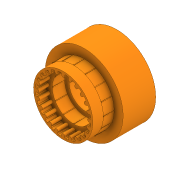
# Autodesk Inventor part: 4th Axis Barrel
Saved by Autodesk Inventor 2020 (Build 240168000, 168)
## iProperties
Created: 2021-06-26
Part Number: 4th Axis Barrel
Material: Generic
Document SubType Name: Modeling
Designer: Coy
Density: 1 g/cm^3
Appearance: Orange
Author: Coy
Autodesk Inventor part; units mm, degrees
ref_plane "YZ Plane" through (0, 0, 0) normal (1, 0, 0) x (0, 1, 0)
ref_plane "XZ Plane" through (0, 0, 0) normal (0, 1, 0) x (-1, 0, 0)
ref_plane "XY Plane" through (0, 0, 0) normal (0, 0, 1) x (1, 0, 0)
sketch "Sketch1" plane through (0, 0, 0) normal (0, 0, 1) x (1, 0, 0)
  circle A0 centre (0, 0) radius 11
  circle A1 centre (0, 0) radius 26
  dimension "d0" = 22
  dimension "d1" = 52
  constraints: 2 centre point, 2 coincident
  measures "d0" diameter of A0
  measures "d1" diameter of A1
extrude "Extrusion1" add sketch "Sketch1" against normal blind 21.75
sketch "Sketch2" plane through (0, 0, 0) normal (0, 0, 1) x (1, 0, 0)
  circle A0 centre (0, 0) radius 14
  circle A1 centre (0, 0) radius 20
  dimension "d4" = 28
  dimension "d5" = 40
  constraints: 2 centre point, 2 coincident
  measures "d4" diameter of A0
  measures "d5" diameter of A1
extrude "Extrusion2" add sketch "Sketch2" along normal blind 7
chamfer "Chamfer2" distance 7 angle 2 1 edges at (-20, 0, 7) measured on face at (-20, 0, 6.5)
sketch "Sketch4" plane through (0, 0, 7) normal (0, 0, 1) x (1, 0, 0)
  circle A0 centre (0, 0) radius 20 construction
  circle A1 centre (0, 0) radius 19.7556 projected
  arc A2 (0.2, 19.999) -> (-0.2, 19.999) centre (0, 20) ccw
  line L0 (-0.2, 19.999) -> (-0.1988, 19.7546)
  line L1 (0.2, 19.999) -> (0.1988, 19.7546)
  arc A3 (-7.4685, 18.5532) -> (-7.8381, 18.4001) centre (-7.6537, 18.4776) ccw
  line L2 (-7.8381, 18.4001) -> (-7.7434, 18.1748)
  line L3 (-7.4685, 18.5532) -> (-7.3761, 18.3269)
  arc A4 (-14, 14.2828) -> (-14.2828, 14) centre (-14.1421, 14.1421) ccw
  line L4 (-14.2828, 14) -> (-14.1091, 13.828)
  line L5 (-14, 14.2828) -> (-13.828, 14.1091)
  arc A5 (-18.4001, 7.8381) -> (-18.5532, 7.4685) centre (-18.4776, 7.6537) ccw
  line L6 (-18.5532, 7.4685) -> (-18.3269, 7.3761)
  line L7 (-18.4001, 7.8381) -> (-18.1748, 7.7434)
  arc A6 (-19.999, 0.2) -> (-19.999, -0.2) centre (-20, 0) ccw
  line L8 (-19.999, -0.2) -> (-19.7546, -0.1988)
  line L9 (-19.999, 0.2) -> (-19.7546, 0.1988)
  arc A7 (-18.5532, -7.4685) -> (-18.4001, -7.8381) centre (-18.4776, -7.6537) ccw
  line L10 (-18.4001, -7.8381) -> (-18.1748, -7.7434)
  line L11 (-18.5532, -7.4685) -> (-18.3269, -7.3761)
  arc A8 (-14.2828, -14) -> (-14, -14.2828) centre (-14.1421, -14.1421) ccw
  line L12 (-14, -14.2828) -> (-13.828, -14.1091)
  line L13 (-14.2828, -14) -> (-14.1091, -13.828)
  arc A9 (-7.8381, -18.4001) -> (-7.4685, -18.5532) centre (-7.6537, -18.4776) ccw
  line L14 (-7.4685, -18.5532) -> (-7.3761, -18.3269)
  line L15 (-7.8381, -18.4001) -> (-7.7434, -18.1748)
  arc A10 (-0.2, -19.999) -> (0.2, -19.999) centre (0, -20) ccw
  line L16 (0.2, -19.999) -> (0.1988, -19.7546)
  line L17 (-0.2, -19.999) -> (-0.1988, -19.7546)
  arc A11 (7.4685, -18.5532) -> (7.8381, -18.4001) centre (7.6537, -18.4776) ccw
  line L18 (7.8381, -18.4001) -> (7.7434, -18.1748)
  line L19 (7.4685, -18.5532) -> (7.3761, -18.3269)
  arc A12 (14, -14.2828) -> (14.2828, -14) centre (14.1421, -14.1421) ccw
  line L20 (14.2828, -14) -> (14.1091, -13.828)
  line L21 (14, -14.2828) -> (13.828, -14.1091)
  arc A13 (18.4001, -7.8381) -> (18.5532, -7.4685) centre (18.4776, -7.6537) ccw
  line L22 (18.5532, -7.4685) -> (18.3269, -7.3761)
  line L23 (18.4001, -7.8381) -> (18.1748, -7.7434)
  arc A14 (19.999, -0.2) -> (19.999, 0.2) centre (20, 0) ccw
  line L24 (19.999, 0.2) -> (19.7546, 0.1988)
  line L25 (19.999, -0.2) -> (19.7546, -0.1988)
  arc A15 (18.5532, 7.4685) -> (18.4001, 7.8381) centre (18.4776, 7.6537) ccw
  line L26 (18.4001, 7.8381) -> (18.1748, 7.7434)
  line L27 (18.5532, 7.4685) -> (18.3269, 7.3761)
  arc A16 (14.2828, 14) -> (14, 14.2828) centre (14.1421, 14.1421) ccw
  line L28 (14, 14.2828) -> (13.828, 14.1091)
  line L29 (14.2828, 14) -> (14.1091, 13.828)
  arc A17 (7.8381, 18.4001) -> (7.4685, 18.5532) centre (7.6537, 18.4776) ccw
  line L30 (7.4685, 18.5532) -> (7.3761, 18.3269)
  line L31 (7.8381, 18.4001) -> (7.7434, 18.1748)
  dimension "d25" = 0.4
  dimension "d28" = 360
  constraints: 64 end point, 35 point on circle, 16 centre point, 2 tangent, 132 other
  measures "d25" diameter of A2
extrude "Extrusion4" add sketch "Sketch4" against normal up to surface (7 mm away) contours A1 L24 A14 L25 | A1 L26 A15 L27 | L22 A13 L23 A1 | A1 L28 A16 L29 | L20 A12 L21 A1 | A1 L30 A17 L31 | L18 A11 L19 A1 | A1 L0 A2 L1 | L16 A10 L17 A1 | A1 L2 A3 L3 | L14 A9 L15 A1 | A1 L4 A4 L5 | L12 A8 L13 A1 | A1 L6 A5 L7 | L10 A7 L11 A1 | A1 L8 A6 L9
sketch "Sketch5" plane through (0, 0, 7) normal (0, 0, 1) x (1, 0, 0)
  arc A0 (7.3761, 18.3269) -> (0.1988, 19.7546) centre (0, 0) ccw projected
  arc A1 (-0.1988, 19.7546) -> (-7.3761, 18.3269) centre (0, 0) ccw projected
  circle A2 centre (0, 0) radius 19.7556
  line L0 (0, 0) -> (0, 34.6201) construction
  line L1 (1.1056, 17.9252) -> (1, 16.2136) construction
  line L2 (-1.1056, 17.9252) -> (-1, 16.2136) construction
  arc A3 (-1.0636, 17.2444) -> (1.0636, 17.2444) centre (0, 17.31) ccw
  line L3 (-1.0636, 17.2444) -> (-1.1056, 17.9252)
  line L4 (1.0636, 17.2444) -> (1.1056, 17.9252)
  arc A4 (1.6859, 18.423) -> (1.1056, 17.9252) centre (1.6374, 17.8924) ccw
  arc A5 (-1.1056, 17.9252) -> (-1.6859, 18.423) centre (-1.6374, 17.8924) ccw
  arc A6 (-5.7073, 17.0283) -> (-6.3967, 17.3589) centre (-6.2125, 16.859) ccw
  line L5 (-5.4905, 16.3816) -> (-5.7073, 17.0283)
  arc A7 (-5.4905, 16.3816) -> (-3.4359, 16.9321) centre (-4.4802, 16.7202) ccw
  line L6 (-3.4359, 16.9321) -> (-3.5715, 17.6006)
  arc A8 (-3.1398, 18.2316) -> (-3.5715, 17.6006) centre (-3.0493, 17.7065) ccw
  arc A9 (-9.9201, 14.9709) -> (-10.6715, 15.1119) centre (-10.3642, 14.6766) ccw
  line L7 (-9.5433, 14.4023) -> (-9.9201, 14.9709)
  arc A10 (-9.5433, 14.4023) -> (-7.7011, 15.4659) centre (-8.655, 14.9909) ccw
  line L8 (-7.7011, 15.4659) -> (-8.0052, 16.0765)
  arc A11 (-7.7515, 16.7978) -> (-8.0052, 16.0765) centre (-7.5282, 16.314) ccw
  arc A12 (-13.4568, 11.8933) -> (-14.2192, 11.8349) centre (-13.8096, 11.4941) ccw
  line L9 (-12.9457, 11.4416) -> (-13.4568, 11.8933)
  arc A13 (-12.9457, 11.4416) -> (-11.4416, 12.9457) centre (-12.24, 12.24) ccw
  line L10 (-11.4416, 12.9457) -> (-11.8933, 13.4568)
  arc A14 (-11.8349, 14.2192) -> (-11.8933, 13.4568) centre (-11.4941, 13.8096) ccw
  arc A15 (-16.0765, 8.0052) -> (-16.7978, 7.7515) centre (-16.314, 7.5282) ccw
  line L11 (-15.4659, 7.7011) -> (-16.0765, 8.0052)
  arc A16 (-15.4659, 7.7011) -> (-14.4023, 9.5433) centre (-14.9909, 8.655) ccw
  line L12 (-14.4023, 9.5433) -> (-14.9709, 9.9201)
  arc A17 (-15.1119, 10.6715) -> (-14.9709, 9.9201) centre (-14.6766, 10.3642) ccw
  arc A18 (-17.6006, 3.5715) -> (-18.2316, 3.1398) centre (-17.7065, 3.0493) ccw
  line L13 (-16.9321, 3.4359) -> (-17.6006, 3.5715)
  arc A19 (-16.9321, 3.4359) -> (-16.3816, 5.4905) centre (-16.7202, 4.4802) ccw
  line L14 (-16.3816, 5.4905) -> (-17.0283, 5.7073)
  arc A20 (-17.3589, 6.3967) -> (-17.0283, 5.7073) centre (-16.859, 6.2125) ccw
  arc A21 (-17.9252, -1.1056) -> (-18.423, -1.6859) centre (-17.8924, -1.6374) ccw
  line L15 (-17.2444, -1.0636) -> (-17.9252, -1.1056)
  arc A22 (-17.2444, -1.0636) -> (-17.2444, 1.0636) centre (-17.31, 0) ccw
  line L16 (-17.2444, 1.0636) -> (-17.9252, 1.1056)
  arc A23 (-18.423, 1.6859) -> (-17.9252, 1.1056) centre (-17.8924, 1.6374) ccw
  arc A24 (-17.0283, -5.7073) -> (-17.3589, -6.3967) centre (-16.859, -6.2125) ccw
  line L17 (-16.3816, -5.4905) -> (-17.0283, -5.7073)
  arc A25 (-16.3816, -5.4905) -> (-16.9321, -3.4359) centre (-16.7202, -4.4802) ccw
  line L18 (-16.9321, -3.4359) -> (-17.6006, -3.5715)
  arc A26 (-18.2316, -3.1398) -> (-17.6006, -3.5715) centre (-17.7065, -3.0493) ccw
  arc A27 (-14.9709, -9.9201) -> (-15.1119, -10.6715) centre (-14.6766, -10.3642) ccw
  line L19 (-14.4023, -9.5433) -> (-14.9709, -9.9201)
  arc A28 (-14.4023, -9.5433) -> (-15.4659, -7.7011) centre (-14.9909, -8.655) ccw
  line L20 (-15.4659, -7.7011) -> (-16.0765, -8.0052)
  arc A29 (-16.7978, -7.7515) -> (-16.0765, -8.0052) centre (-16.314, -7.5282) ccw
  arc A30 (-11.8933, -13.4568) -> (-11.8349, -14.2192) centre (-11.4941, -13.8096) ccw
  line L21 (-11.4416, -12.9457) -> (-11.8933, -13.4568)
  arc A31 (-11.4416, -12.9457) -> (-12.9457, -11.4416) centre (-12.24, -12.24) ccw
  line L22 (-12.9457, -11.4416) -> (-13.4568, -11.8933)
  arc A32 (-14.2192, -11.8349) -> (-13.4568, -11.8933) centre (-13.8096, -11.4941) ccw
  arc A33 (-8.0052, -16.0765) -> (-7.7515, -16.7978) centre (-7.5282, -16.314) ccw
  line L23 (-7.7011, -15.4659) -> (-8.0052, -16.0765)
  arc A34 (-7.7011, -15.4659) -> (-9.5433, -14.4023) centre (-8.655, -14.9909) ccw
  line L24 (-9.5433, -14.4023) -> (-9.9201, -14.9709)
  arc A35 (-10.6715, -15.1119) -> (-9.9201, -14.9709) centre (-10.3642, -14.6766) ccw
  arc A36 (-3.5715, -17.6006) -> (-3.1398, -18.2316) centre (-3.0493, -17.7065) ccw
  line L25 (-3.4359, -16.9321) -> (-3.5715, -17.6006)
  arc A37 (-3.4359, -16.9321) -> (-5.4905, -16.3816) centre (-4.4802, -16.7202) ccw
  line L26 (-5.4905, -16.3816) -> (-5.7073, -17.0283)
  arc A38 (-6.3967, -17.3589) -> (-5.7073, -17.0283) centre (-6.2125, -16.859) ccw
  arc A39 (1.1056, -17.9252) -> (1.6859, -18.423) centre (1.6374, -17.8924) ccw
  line L27 (1.0636, -17.2444) -> (1.1056, -17.9252)
  arc A40 (1.0636, -17.2444) -> (-1.0636, -17.2444) centre (0, -17.31) ccw
  line L28 (-1.0636, -17.2444) -> (-1.1056, -17.9252)
  arc A41 (-1.6859, -18.423) -> (-1.1056, -17.9252) centre (-1.6374, -17.8924) ccw
  arc A42 (5.7073, -17.0283) -> (6.3967, -17.3589) centre (6.2125, -16.859) ccw
  line L29 (5.4905, -16.3816) -> (5.7073, -17.0283)
  arc A43 (5.4905, -16.3816) -> (3.4359, -16.9321) centre (4.4802, -16.7202) ccw
  line L30 (3.4359, -16.9321) -> (3.5715, -17.6006)
  arc A44 (3.1398, -18.2316) -> (3.5715, -17.6006) centre (3.0493, -17.7065) ccw
  arc A45 (9.9201, -14.9709) -> (10.6715, -15.1119) centre (10.3642, -14.6766) ccw
  line L31 (9.5433, -14.4023) -> (9.9201, -14.9709)
  arc A46 (9.5433, -14.4023) -> (7.7011, -15.4659) centre (8.655, -14.9909) ccw
  line L32 (7.7011, -15.4659) -> (8.0052, -16.0765)
  arc A47 (7.7515, -16.7978) -> (8.0052, -16.0765) centre (7.5282, -16.314) ccw
  arc A48 (13.4568, -11.8933) -> (14.2192, -11.8349) centre (13.8096, -11.4941) ccw
  line L33 (12.9457, -11.4416) -> (13.4568, -11.8933)
  arc A49 (12.9457, -11.4416) -> (11.4416, -12.9457) centre (12.24, -12.24) ccw
  line L34 (11.4416, -12.9457) -> (11.8933, -13.4568)
  arc A50 (11.8349, -14.2192) -> (11.8933, -13.4568) centre (11.4941, -13.8096) ccw
  arc A51 (16.0765, -8.0052) -> (16.7978, -7.7515) centre (16.314, -7.5282) ccw
  line L35 (15.4659, -7.7011) -> (16.0765, -8.0052)
  arc A52 (15.4659, -7.7011) -> (14.4023, -9.5433) centre (14.9909, -8.655) ccw
  line L36 (14.4023, -9.5433) -> (14.9709, -9.9201)
  arc A53 (15.1119, -10.6715) -> (14.9709, -9.9201) centre (14.6766, -10.3642) ccw
  arc A54 (17.6006, -3.5715) -> (18.2316, -3.1398) centre (17.7065, -3.0493) ccw
  line L37 (16.9321, -3.4359) -> (17.6006, -3.5715)
  arc A55 (16.9321, -3.4359) -> (16.3816, -5.4905) centre (16.7202, -4.4802) ccw
  line L38 (16.3816, -5.4905) -> (17.0283, -5.7073)
  arc A56 (17.3589, -6.3967) -> (17.0283, -5.7073) centre (16.859, -6.2125) ccw
  arc A57 (17.9252, 1.1056) -> (18.423, 1.6859) centre (17.8924, 1.6374) ccw
  line L39 (17.2444, 1.0636) -> (17.9252, 1.1056)
  arc A58 (17.2444, 1.0636) -> (17.2444, -1.0636) centre (17.31, 0) ccw
  line L40 (17.2444, -1.0636) -> (17.9252, -1.1056)
  arc A59 (18.423, -1.6859) -> (17.9252, -1.1056) centre (17.8924, -1.6374) ccw
  arc A60 (17.0283, 5.7073) -> (17.3589, 6.3967) centre (16.859, 6.2125) ccw
  line L41 (16.3816, 5.4905) -> (17.0283, 5.7073)
  arc A61 (16.3816, 5.4905) -> (16.9321, 3.4359) centre (16.7202, 4.4802) ccw
  line L42 (16.9321, 3.4359) -> (17.6006, 3.5715)
  arc A62 (18.2316, 3.1398) -> (17.6006, 3.5715) centre (17.7065, 3.0493) ccw
  arc A63 (14.9709, 9.9201) -> (15.1119, 10.6715) centre (14.6766, 10.3642) ccw
  line L43 (14.4023, 9.5433) -> (14.9709, 9.9201)
  arc A64 (14.4023, 9.5433) -> (15.4659, 7.7011) centre (14.9909, 8.655) ccw
  line L44 (15.4659, 7.7011) -> (16.0765, 8.0052)
  arc A65 (16.7978, 7.7515) -> (16.0765, 8.0052) centre (16.314, 7.5282) ccw
  arc A66 (11.8933, 13.4568) -> (11.8349, 14.2192) centre (11.4941, 13.8096) ccw
  line L45 (11.4416, 12.9457) -> (11.8933, 13.4568)
  arc A67 (11.4416, 12.9457) -> (12.9457, 11.4416) centre (12.24, 12.24) ccw
  line L46 (12.9457, 11.4416) -> (13.4568, 11.8933)
  arc A68 (14.2192, 11.8349) -> (13.4568, 11.8933) centre (13.8096, 11.4941) ccw
  arc A69 (8.0052, 16.0765) -> (7.7515, 16.7978) centre (7.5282, 16.314) ccw
  line L47 (7.7011, 15.4659) -> (8.0052, 16.0765)
  arc A70 (7.7011, 15.4659) -> (9.5433, 14.4023) centre (8.655, 14.9909) ccw
  line L48 (9.5433, 14.4023) -> (9.9201, 14.9709)
  arc A71 (10.6715, 15.1119) -> (9.9201, 14.9709) centre (10.3642, 14.6766) ccw
  arc A72 (3.5715, 17.6006) -> (3.1398, 18.2316) centre (3.0493, 17.7065) ccw
  line L49 (3.4359, 16.9321) -> (3.5715, 17.6006)
  arc A73 (3.4359, 16.9321) -> (5.4905, 16.3816) centre (4.4802, 16.7202) ccw
  line L50 (5.4905, 16.3816) -> (5.7073, 17.0283)
  arc A74 (6.3967, 17.3589) -> (5.7073, 17.0283) centre (6.2125, 16.859) ccw
  arc A75 (-1.6859, 18.423) -> (-3.1398, 18.2316) centre (0, 0) ccw
  arc A76 (-6.3967, 17.3589) -> (-7.7515, 16.7978) centre (0, 0) ccw
  arc A77 (-10.6715, 15.1119) -> (-11.8349, 14.2192) centre (0, 0) ccw
  arc A78 (-14.2192, 11.8349) -> (-15.1119, 10.6715) centre (0, 0) ccw
  arc A79 (-16.7978, 7.7515) -> (-17.3589, 6.3967) centre (0, 0) ccw
  arc A80 (-18.2316, 3.1398) -> (-18.423, 1.6859) centre (0, 0) ccw
  arc A81 (-18.423, -1.6859) -> (-18.2316, -3.1398) centre (0, 0) ccw
  arc A82 (-17.3589, -6.3967) -> (-16.7978, -7.7515) centre (0, 0) ccw
  arc A83 (-15.1119, -10.6715) -> (-14.2192, -11.8349) centre (0, 0) ccw
  arc A84 (-11.8349, -14.2192) -> (-10.6715, -15.1119) centre (0, 0) ccw
  arc A85 (-7.7515, -16.7978) -> (-6.3967, -17.3589) centre (0, 0) ccw
  arc A86 (-3.1398, -18.2316) -> (-1.6859, -18.423) centre (0, 0) ccw
  arc A87 (1.6859, -18.423) -> (3.1398, -18.2316) centre (0, 0) ccw
  arc A88 (6.3967, -17.3589) -> (7.7515, -16.7978) centre (0, 0) ccw
  arc A89 (10.6715, -15.1119) -> (11.8349, -14.2192) centre (0, 0) ccw
  arc A90 (14.2192, -11.8349) -> (15.1119, -10.6715) centre (0, 0) ccw
  arc A91 (16.7978, -7.7515) -> (17.3589, -6.3967) centre (0, 0) ccw
  arc A92 (18.2316, -3.1398) -> (18.423, -1.6859) centre (0, 0) ccw
  arc A93 (18.423, 1.6859) -> (18.2316, 3.1398) centre (0, 0) ccw
  arc A94 (17.3589, 6.3967) -> (16.7978, 7.7515) centre (0, 0) ccw
  arc A95 (15.1119, 10.6715) -> (14.2192, 11.8349) centre (0, 0) ccw
  arc A96 (11.8349, 14.2192) -> (10.6715, 15.1119) centre (0, 0) ccw
  arc A97 (7.7515, 16.7978) -> (6.3967, 17.3589) centre (0, 0) ccw
  arc A98 (3.1398, 18.2316) -> (1.6859, 18.423) centre (0, 0) ccw
  circle A99 centre (0, 0) radius 16 construction
  point P0 (0.1988, 19.7546)
  point P1 (-7.3761, 18.3269)
  point P2 (7.3761, 18.3269)
  dimension "d33" = 1
  dimension "d38" = 1
  dimension "d40" = 1.0656
  dimension "d41" = 1.0656
  dimension "d42" = 1.0656
  dimension "d45" = 360
  dimension "d49" = 32
  constraints: 192 point on circle, 102 end point, 97 centre point, 4 coincident, 3 tangent, 2 line through centre, 2 point on line, 1 midpoint, 1 vertical, 340 other
  measures "d33" distance from line of L0 L2.end
  measures "d38" distance from line of L0 L1.end
  measures "d40" radius of A3
  measures "d41" diameter of A5
  measures "d42" diameter of A4
  measures "d49" diameter of A99
extrude "Extrusion5" add sketch "Sketch5" along normal blind 7
sketch "Sketch8" plane through (0, 0, 0) normal (0, 0, 1) x (1, 0, 0)
  circle A0 centre (0, 0) radius 14 projected
  circle A1 centre (0, 0) radius 11 projected
extrude "Extrusion7" cut sketch "Sketch8" against normal blind 1
chamfer "Chamfer4" distance 8 angle 2 1 edges at (-14, 0, 7) measured on face at (-14, 0, 6.5)
sketch "Sketch10" plane through (0, 0, 7) normal (0, 0, 1) x (1, 0, 0)
  circle A0 centre (0, 0) radius 14 construction
  circle A1 centre (0, 0) radius 14.2794 projected
  arc A2 (-0.2, 13.9986) -> (0.2, 13.9986) centre (0, 14) ccw
  line L0 (0.204, 14.2779) -> (0.2, 13.9971)
  line L1 (-0.204, 14.2779) -> (-0.2, 13.9971)
  line L2 (-7.3156, 12.263) -> (-7.1718, 12.0219)
  arc A3 (-7.1725, 12.0231) -> (-6.8261, 12.2231) centre (-7, 12.1244) ccw
  line L3 (-6.9623, 12.467) -> (-6.8254, 12.2219)
  line L4 (-12.467, 6.9623) -> (-12.2219, 6.8254)
  arc A4 (-12.2231, 6.8261) -> (-12.0231, 7.1725) centre (-12.1244, 7) ccw
  line L5 (-12.263, 7.3156) -> (-12.0219, 7.1718)
  line L6 (-14.2779, -0.204) -> (-13.9971, -0.2)
  arc A5 (-13.9986, -0.2) -> (-13.9986, 0.2) centre (-14, 0) ccw
  line L7 (-14.2779, 0.204) -> (-13.9971, 0.2)
  line L8 (-12.263, -7.3156) -> (-12.0219, -7.1718)
  arc A6 (-12.0231, -7.1725) -> (-12.2231, -6.8261) centre (-12.1244, -7) ccw
  line L9 (-12.467, -6.9623) -> (-12.2219, -6.8254)
  line L10 (-6.9623, -12.467) -> (-6.8254, -12.2219)
  arc A7 (-6.8261, -12.2231) -> (-7.1725, -12.0231) centre (-7, -12.1244) ccw
  line L11 (-7.3156, -12.263) -> (-7.1718, -12.0219)
  line L12 (0.204, -14.2779) -> (0.2, -13.9971)
  arc A8 (0.2, -13.9986) -> (-0.2, -13.9986) centre (0, -14) ccw
  line L13 (-0.204, -14.2779) -> (-0.2, -13.9971)
  line L14 (7.3156, -12.263) -> (7.1718, -12.0219)
  arc A9 (7.1725, -12.0231) -> (6.8261, -12.2231) centre (7, -12.1244) ccw
  line L15 (6.9623, -12.467) -> (6.8254, -12.2219)
  line L16 (12.467, -6.9623) -> (12.2219, -6.8254)
  arc A10 (12.2231, -6.8261) -> (12.0231, -7.1725) centre (12.1244, -7) ccw
  line L17 (12.263, -7.3156) -> (12.0219, -7.1718)
  line L18 (14.2779, 0.204) -> (13.9971, 0.2)
  arc A11 (13.9986, 0.2) -> (13.9986, -0.2) centre (14, 0) ccw
  line L19 (14.2779, -0.204) -> (13.9971, -0.2)
  line L20 (12.263, 7.3156) -> (12.0219, 7.1718)
  arc A12 (12.0231, 7.1725) -> (12.2231, 6.8261) centre (12.1244, 7) ccw
  line L21 (12.467, 6.9623) -> (12.2219, 6.8254)
  line L22 (6.9623, 12.467) -> (6.8254, 12.2219)
  arc A13 (6.8261, 12.2231) -> (7.1725, 12.0231) centre (7, 12.1244) ccw
  line L23 (7.3156, 12.263) -> (7.1718, 12.0219)
  point P0 (13.9986, -0.2)
  point P1 (12.0231, -7.1725)
  point P2 (6.8261, -12.2231)
  point P3 (-0.2, -13.9986)
  point P4 (-7.1725, -12.0231)
  point P5 (7.1725, 12.0231)
  point P6 (0.2, 13.9986)
  point P7 (-12.0231, 7.1725)
  point P8 (-13.9986, 0.2)
  dimension "d67" = 0.4
  dimension "d70" = 360
  constraints: 53 point on circle, 48 end point, 12 centre point, 2 line through centre, 2 tangent, 122 other
  measures "d67" diameter of A2
extrude "Extrusion8" add sketch "Sketch10" against normal up to surface (8 mm away) contours A1 L19 A11 L18 | L21 A12 L20 A1 | A1 L17 A10 L16 | L23 A13 L22 A1 | A1 L15 A9 L14 | L0 A2 L1 A1 | A1 L13 A8 L12 | L3 A3 L2 A1 | A1 L11 A7 L10 | L5 A4 L4 A1 | A1 L9 A6 L8 | L7 A5 L6 A1
equation "\"d41\" = d40"
equation "\"d42\" = d40"
body "Solid1"
